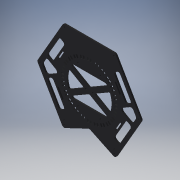
# Autodesk Inventor part: Bottom Plate
Saved by Autodesk Inventor 2017 (Build 210142000, 142)
## iProperties
Created: 2016-10-01
Part Number: Bottom Plate
Material: PVC, Unplasticized
Document SubType Name: Modeling
Designer: James Yelland
Density: 1.29 g/cm^3
Appearance: Smooth - White
Mass: 43.6601 g
Surface Area: 401.333 cm^2
Volume: 33.8451 cm^3
Author: James Yelland
Autodesk Inventor part; units mm, degrees
ref_plane "YZ Plane" through (0, 0, 0) normal (1, 0, 0) x (0, 1, 0)
ref_plane "XZ Plane" through (0, 0, 0) normal (0, 1, 0) x (-1, 0, 0)
ref_plane "XY Plane" through (0, 0, 0) normal (0, 0, 1) x (1, 0, 0)
sketch "Sketch1" plane through (0, 0, 0) normal (0, 1, 0) x (-1, 0, 0)
  line L0 (72.6878, -41.9663) -> (62.1878, -60.1529)
  line L1 (72.6878, -41.9663) -> (83.1878, -23.7798)
  line L2 (81.7237, -18.3157) -> (77.3936, -15.8157)
  line L3 (71.9295, -17.2797) -> (50.9295, -53.6529)
  line L4 (52.3936, -59.117) -> (56.7237, -61.617)
  arc A0 (56.7237, -61.617) -> (62.1878, -60.1529) centre (58.7237, -58.1529) ccw
  arc A1 (50.9295, -53.6529) -> (52.3936, -59.117) centre (54.3936, -55.6529) ccw
  arc A2 (77.3936, -15.8157) -> (71.9295, -17.2797) centre (75.3936, -19.2798) ccw
  arc A3 (83.1878, -23.7798) -> (81.7237, -18.3157) centre (79.7237, -21.7798) ccw
  line L5 (-72.6878, -41.9663) -> (-83.1878, -23.7798)
  line L6 (-72.6878, -41.9663) -> (-62.1878, -60.1529)
  line L7 (-56.7237, -61.617) -> (-52.3936, -59.117)
  line L8 (-50.9295, -53.6529) -> (-71.9294, -17.28)
  line L9 (-77.3936, -15.8157) -> (-81.7237, -18.3157)
  arc A4 (-81.7237, -18.3157) -> (-83.1878, -23.7798) centre (-79.7237, -21.7798) ccw
  arc A5 (-71.9294, -17.28) -> (-77.3936, -15.8157) centre (-75.3936, -19.2798) ccw
  arc A6 (-52.3936, -59.117) -> (-50.9295, -53.6529) centre (-54.3936, -55.6529) ccw
  arc A7 (-62.1878, -60.1529) -> (-56.7237, -61.617) centre (-58.7237, -58.1529) ccw
  line L10 (103.5566, -2.5) -> (54.8095, -86.9325)
  line L11 (-54.8095, -86.9325) -> (-103.5566, -2.5)
  line L12 (-103.5566, 2.5) -> (-53.9434, 88.4327)
  line L13 (-49.6132, 90.9327) -> (49.6132, 90.9327)
  line L14 (53.9434, 88.4327) -> (103.5566, 2.5)
  line L15 (2.1497, -66.9563) -> (48.3297, -88.9468)
  line L16 (-2.1497, -66.9563) -> (-48.3297, -88.9468)
  arc A8 (48.3297, -88.9468) -> (54.8095, -86.9325) centre (50.4794, -84.4325) ccw
  arc A9 (2.1497, -66.9563) -> (-2.1497, -66.9563) centre (0, -71.4706) ccw
  arc A10 (-54.8095, -86.9325) -> (-48.3297, -88.9468) centre (-50.4794, -84.4325) ccw
  arc A11 (-103.5566, 2.5) -> (-103.5566, -2.5) centre (-99.2265, 0) ccw
  arc A12 (-49.6132, 90.9327) -> (-53.9434, 88.4327) centre (-49.6132, 85.9327) ccw
  arc A13 (53.9434, 88.4327) -> (49.6132, 90.9327) centre (49.6132, 85.9327) ccw
  arc A14 (103.5566, -2.5) -> (103.5566, 2.5) centre (99.2265, 0) ccw
  circle A15 centre (49.6132, 85.9327) radius 1.6
  circle A16 centre (-49.6132, 85.9327) radius 1.6
  circle A17 centre (-99.2265, 0) radius 1.6
  circle A18 centre (99.2265, 0) radius 1.6
  arc A19 (-88.75, -10.8253) -> (-81.9199, -12.6554) centre (-84.4199, -8.3253) ccw
  arc A20 (-93.5566, 2.5) -> (-93.5566, -2.5) centre (-89.2265, 0) ccw
  arc A21 (81.9199, -12.6554) -> (88.75, -10.8253) centre (84.4199, -8.3253) ccw
  arc A22 (93.5566, -2.5) -> (93.5566, 2.5) centre (89.2265, 0) ccw
  line L17 (1.5, -53.75) -> (1.5, -56.75)
  line L18 (1.5, -56.75) -> (4.5, -56.75)
  line L19 (4.5, -56.75) -> (4.5, -50.75)
  line L20 (4.5, -50.75) -> (1.5, -50.75)
  line L21 (1.5, -50.75) -> (1.5, -53.75)
  line L22 (-1.5, -53.75) -> (-1.5, -56.75)
  line L23 (-1.5, -56.75) -> (-4.5, -56.75)
  line L24 (-1.5, -53.75) -> (-1.5, -53.75)
  line L25 (-1.5, -53.75) -> (-1.5, -50.75)
  line L26 (-1.5, -50.75) -> (-4.5, -50.75)
  line L27 (-4.5, -56.75) -> (-4.5, -50.75)
  line L28 (15.3604, -51.5303) -> (16.1369, -54.4281)
  line L29 (16.1369, -54.4281) -> (19.0346, -53.6516)
  line L30 (19.0346, -53.6516) -> (17.4817, -47.856)
  line L31 (17.4817, -47.856) -> (14.584, -48.6325)
  line L32 (14.584, -48.6325) -> (15.3604, -51.5303)
  line L33 (12.4626, -52.3067) -> (13.2391, -55.2045)
  line L34 (13.2391, -55.2045) -> (10.3413, -55.981)
  line L35 (12.4626, -52.3067) -> (11.6862, -49.409)
  line L36 (11.6862, -49.409) -> (8.7884, -50.1854)
  line L37 (10.3413, -55.981) -> (8.7884, -50.1854)
  line L38 (28.174, -45.7989) -> (29.674, -48.3969)
  line L39 (29.674, -48.3969) -> (32.2721, -46.8969)
  line L40 (32.2721, -46.8969) -> (29.2721, -41.7008)
  line L41 (29.2721, -41.7008) -> (26.674, -43.2008)
  line L42 (26.674, -43.2008) -> (28.174, -45.7989)
  line L43 (25.576, -47.2989) -> (27.076, -49.8969)
  line L44 (27.076, -49.8969) -> (24.4779, -51.3969)
  line L45 (25.576, -47.2989) -> (24.076, -44.7008)
  line L46 (24.076, -44.7008) -> (21.4779, -46.2008)
  line L47 (24.4779, -51.3969) -> (21.4779, -46.2008)
  line L48 (39.0676, -36.9463) -> (41.189, -39.0676)
  line L49 (41.189, -39.0676) -> (43.3103, -36.9463)
  line L50 (43.3103, -36.9463) -> (39.0676, -32.7037)
  line L51 (39.0676, -32.7037) -> (36.9463, -34.825)
  line L52 (36.9463, -34.825) -> (39.0676, -36.9463)
  line L53 (36.9463, -39.0676) -> (39.0676, -41.189)
  line L54 (39.0676, -41.189) -> (36.9463, -43.3103)
  line L55 (36.9463, -39.0676) -> (34.825, -36.9463)
  line L56 (34.825, -36.9463) -> (32.7037, -39.0676)
  line L57 (36.9463, -43.3103) -> (32.7037, -39.0676)
  line L58 (47.2989, -25.576) -> (49.8969, -27.076)
  line L59 (49.8969, -27.076) -> (51.3969, -24.4779)
  line L60 (51.3969, -24.4779) -> (46.2008, -21.4779)
  line L61 (46.2008, -21.4779) -> (44.7008, -24.076)
  line L62 (44.7008, -24.076) -> (47.2989, -25.576)
  line L63 (45.7989, -28.174) -> (48.3969, -29.674)
  line L64 (48.3969, -29.674) -> (46.8969, -32.2721)
  line L65 (45.7989, -28.174) -> (43.2008, -26.674)
  line L66 (43.2008, -26.674) -> (41.7008, -29.2721)
  line L67 (46.8969, -32.2721) -> (41.7008, -29.2721)
  line L68 (52.3067, -12.4626) -> (55.2045, -13.2391)
  line L69 (55.2045, -13.2391) -> (55.981, -10.3413)
  line L70 (55.981, -10.3413) -> (50.1854, -8.7884)
  line L71 (50.1854, -8.7884) -> (49.409, -11.6862)
  line L72 (49.409, -11.6862) -> (52.3067, -12.4626)
  line L73 (51.5303, -15.3604) -> (54.4281, -16.1369)
  line L74 (54.4281, -16.1369) -> (53.6516, -19.0346)
  line L75 (51.5303, -15.3604) -> (48.6325, -14.584)
  line L76 (48.6325, -14.584) -> (47.856, -17.4817)
  line L77 (53.6516, -19.0346) -> (47.856, -17.4817)
  line L78 (53.75, 1.5) -> (56.75, 1.5)
  line L79 (56.75, 1.5) -> (56.75, 4.5)
  line L80 (56.75, 4.5) -> (50.75, 4.5)
  line L81 (50.75, 4.5) -> (50.75, 1.5)
  line L82 (50.75, 1.5) -> (53.75, 1.5)
  line L83 (53.75, -1.5) -> (56.75, -1.5)
  line L84 (56.75, -1.5) -> (56.75, -4.5)
  line L85 (53.75, -1.5) -> (50.75, -1.5)
  line L86 (50.75, -1.5) -> (50.75, -4.5)
  line L87 (56.75, -4.5) -> (50.75, -4.5)
  line L88 (51.5303, 15.3604) -> (54.4281, 16.1369)
  line L89 (54.4281, 16.1369) -> (53.6516, 19.0346)
  line L90 (53.6516, 19.0346) -> (47.856, 17.4817)
  line L91 (47.856, 17.4817) -> (48.6325, 14.584)
  line L92 (48.6325, 14.584) -> (51.5303, 15.3604)
  line L93 (52.3067, 12.4626) -> (55.2045, 13.2391)
  line L94 (55.2045, 13.2391) -> (55.981, 10.3413)
  line L95 (52.3067, 12.4626) -> (49.409, 11.6862)
  line L96 (49.409, 11.6862) -> (50.1854, 8.7884)
  line L97 (55.981, 10.3413) -> (50.1854, 8.7884)
  line L98 (45.7989, 28.174) -> (48.3969, 29.674)
  line L99 (48.3969, 29.674) -> (46.8969, 32.2721)
  line L100 (46.8969, 32.2721) -> (41.7008, 29.2721)
  line L101 (41.7008, 29.2721) -> (43.2008, 26.674)
  line L102 (43.2008, 26.674) -> (45.7989, 28.174)
  line L103 (47.2989, 25.576) -> (49.8969, 27.076)
  line L104 (49.8969, 27.076) -> (51.3969, 24.4779)
  line L105 (47.2989, 25.576) -> (44.7008, 24.076)
  line L106 (44.7008, 24.076) -> (46.2008, 21.4779)
  line L107 (51.3969, 24.4779) -> (46.2008, 21.4779)
  line L108 (36.9463, 39.0676) -> (39.0676, 41.189)
  line L109 (39.0676, 41.189) -> (36.9463, 43.3103)
  line L110 (36.9463, 43.3103) -> (32.7037, 39.0676)
  line L111 (32.7037, 39.0676) -> (34.825, 36.9463)
  line L112 (34.825, 36.9463) -> (36.9463, 39.0676)
  line L113 (39.0676, 36.9463) -> (41.189, 39.0676)
  line L114 (41.189, 39.0676) -> (43.3103, 36.9463)
  line L115 (39.0676, 36.9463) -> (36.9463, 34.825)
  line L116 (36.9463, 34.825) -> (39.0676, 32.7037)
  line L117 (43.3103, 36.9463) -> (39.0676, 32.7037)
  line L118 (25.576, 47.2989) -> (27.076, 49.8969)
  line L119 (27.076, 49.8969) -> (24.4779, 51.3969)
  line L120 (24.4779, 51.3969) -> (21.4779, 46.2008)
  line L121 (21.4779, 46.2008) -> (24.076, 44.7008)
  line L122 (24.076, 44.7008) -> (25.576, 47.2989)
  line L123 (28.174, 45.7989) -> (29.674, 48.3969)
  line L124 (29.674, 48.3969) -> (32.2721, 46.8969)
  line L125 (28.174, 45.7989) -> (26.674, 43.2008)
  line L126 (26.674, 43.2008) -> (29.2721, 41.7008)
  line L127 (32.2721, 46.8969) -> (29.2721, 41.7008)
  line L128 (12.4626, 52.3067) -> (13.2391, 55.2045)
  line L129 (13.2391, 55.2045) -> (10.3413, 55.981)
  line L130 (10.3413, 55.981) -> (8.7884, 50.1854)
  line L131 (8.7884, 50.1854) -> (11.6862, 49.409)
  line L132 (11.6862, 49.409) -> (12.4626, 52.3067)
  line L133 (15.3604, 51.5303) -> (16.1369, 54.4281)
  line L134 (16.1369, 54.4281) -> (19.0346, 53.6516)
  line L135 (15.3604, 51.5303) -> (14.584, 48.6325)
  line L136 (14.584, 48.6325) -> (17.4817, 47.856)
  line L137 (19.0346, 53.6516) -> (17.4817, 47.856)
  line L138 (-1.5, 53.75) -> (-1.5, 56.75)
  line L139 (-1.5, 56.75) -> (-4.5, 56.75)
  line L140 (-4.5, 56.75) -> (-4.5, 50.75)
  line L141 (-4.5, 50.75) -> (-1.5, 50.75)
  line L142 (-1.5, 50.75) -> (-1.5, 53.75)
  line L143 (1.5, 53.75) -> (1.5, 56.75)
  line L144 (1.5, 56.75) -> (4.5, 56.75)
  line L145 (1.5, 53.75) -> (1.5, 50.75)
  line L146 (1.5, 50.75) -> (4.5, 50.75)
  line L147 (4.5, 56.75) -> (4.5, 50.75)
  line L148 (-15.3604, 51.5303) -> (-16.1369, 54.4281)
  line L149 (-16.1369, 54.4281) -> (-19.0346, 53.6516)
  line L150 (-19.0346, 53.6516) -> (-17.4817, 47.856)
  line L151 (-17.4817, 47.856) -> (-14.584, 48.6325)
  line L152 (-14.584, 48.6325) -> (-15.3604, 51.5303)
  line L153 (-12.4626, 52.3067) -> (-13.2391, 55.2045)
  line L154 (-13.2391, 55.2045) -> (-10.3413, 55.981)
  line L155 (-12.4626, 52.3067) -> (-11.6862, 49.409)
  line L156 (-11.6862, 49.409) -> (-8.7884, 50.1854)
  line L157 (-10.3413, 55.981) -> (-8.7884, 50.1854)
  line L158 (-28.174, 45.7989) -> (-29.674, 48.3969)
  line L159 (-29.674, 48.3969) -> (-32.2721, 46.8969)
  line L160 (-32.2721, 46.8969) -> (-29.2721, 41.7008)
  line L161 (-29.2721, 41.7008) -> (-26.674, 43.2008)
  line L162 (-26.674, 43.2008) -> (-28.174, 45.7989)
  line L163 (-25.576, 47.2989) -> (-27.076, 49.8969)
  line L164 (-27.076, 49.8969) -> (-24.4779, 51.3969)
  line L165 (-25.576, 47.2989) -> (-24.076, 44.7008)
  line L166 (-24.076, 44.7008) -> (-21.4779, 46.2008)
  line L167 (-24.4779, 51.3969) -> (-21.4779, 46.2008)
  line L168 (-39.0676, 36.9463) -> (-41.189, 39.0676)
  line L169 (-41.189, 39.0676) -> (-43.3103, 36.9463)
  line L170 (-43.3103, 36.9463) -> (-39.0676, 32.7037)
  line L171 (-39.0676, 32.7037) -> (-36.9463, 34.825)
  line L172 (-36.9463, 34.825) -> (-39.0676, 36.9463)
  line L173 (-36.9463, 39.0676) -> (-39.0676, 41.189)
  line L174 (-39.0676, 41.189) -> (-36.9463, 43.3103)
  line L175 (-36.9463, 39.0676) -> (-34.825, 36.9463)
  line L176 (-34.825, 36.9463) -> (-32.7037, 39.0676)
  line L177 (-36.9463, 43.3103) -> (-32.7037, 39.0676)
  line L178 (-47.2989, 25.576) -> (-49.8969, 27.076)
  line L179 (-49.8969, 27.076) -> (-51.3969, 24.4779)
  line L180 (-51.3969, 24.4779) -> (-46.2008, 21.4779)
  line L181 (-46.2008, 21.4779) -> (-44.7008, 24.076)
  line L182 (-44.7008, 24.076) -> (-47.2989, 25.576)
  line L183 (-45.7989, 28.174) -> (-48.3969, 29.674)
  line L184 (-48.3969, 29.674) -> (-46.8969, 32.2721)
  line L185 (-45.7989, 28.174) -> (-43.2008, 26.674)
  line L186 (-43.2008, 26.674) -> (-41.7008, 29.2721)
  line L187 (-46.8969, 32.2721) -> (-41.7008, 29.2721)
  line L188 (-52.3067, 12.4626) -> (-55.2045, 13.2391)
  line L189 (-55.2045, 13.2391) -> (-55.981, 10.3413)
  line L190 (-55.981, 10.3413) -> (-50.1854, 8.7884)
  line L191 (-50.1854, 8.7884) -> (-49.409, 11.6862)
  line L192 (-49.409, 11.6862) -> (-52.3067, 12.4626)
  line L193 (-51.5303, 15.3604) -> (-54.4281, 16.1369)
  line L194 (-54.4281, 16.1369) -> (-53.6516, 19.0346)
  line L195 (-51.5303, 15.3604) -> (-48.6325, 14.584)
  line L196 (-48.6325, 14.584) -> (-47.856, 17.4817)
  line L197 (-53.6516, 19.0346) -> (-47.856, 17.4817)
  line L198 (-53.75, -1.5) -> (-56.75, -1.5)
  line L199 (-56.75, -1.5) -> (-56.75, -4.5)
  line L200 (-56.75, -4.5) -> (-50.75, -4.5)
  line L201 (-50.75, -4.5) -> (-50.75, -1.5)
  line L202 (-50.75, -1.5) -> (-53.75, -1.5)
  line L203 (-53.75, 1.5) -> (-56.75, 1.5)
  line L204 (-56.75, 1.5) -> (-56.75, 4.5)
  line L205 (-53.75, 1.5) -> (-50.75, 1.5)
  line L206 (-50.75, 1.5) -> (-50.75, 4.5)
  line L207 (-56.75, 4.5) -> (-50.75, 4.5)
  line L208 (-51.5303, -15.3604) -> (-54.4281, -16.1369)
  line L209 (-54.4281, -16.1369) -> (-53.6516, -19.0346)
  line L210 (-53.6516, -19.0346) -> (-47.856, -17.4817)
  line L211 (-47.856, -17.4817) -> (-48.6325, -14.584)
  line L212 (-48.6325, -14.584) -> (-51.5303, -15.3604)
  line L213 (-52.3067, -12.4626) -> (-55.2045, -13.2391)
  line L214 (-55.2045, -13.2391) -> (-55.981, -10.3413)
  line L215 (-52.3067, -12.4626) -> (-49.409, -11.6862)
  line L216 (-49.409, -11.6862) -> (-50.1854, -8.7884)
  line L217 (-55.981, -10.3413) -> (-50.1854, -8.7884)
  line L218 (-45.7989, -28.174) -> (-48.3969, -29.674)
  line L219 (-48.3969, -29.674) -> (-46.8969, -32.2721)
  line L220 (-46.8969, -32.2721) -> (-41.7008, -29.2721)
  line L221 (-41.7008, -29.2721) -> (-43.2008, -26.674)
  line L222 (-43.2008, -26.674) -> (-45.7989, -28.174)
  line L223 (-47.2989, -25.576) -> (-49.8969, -27.076)
  line L224 (-49.8969, -27.076) -> (-51.3969, -24.4779)
  line L225 (-47.2989, -25.576) -> (-44.7008, -24.076)
  line L226 (-44.7008, -24.076) -> (-46.2008, -21.4779)
  line L227 (-51.3969, -24.4779) -> (-46.2008, -21.4779)
  line L228 (-36.9463, -39.0676) -> (-39.0676, -41.189)
  line L229 (-39.0676, -41.189) -> (-36.9463, -43.3103)
  line L230 (-36.9463, -43.3103) -> (-32.7037, -39.0676)
  line L231 (-32.7037, -39.0676) -> (-34.825, -36.9463)
  line L232 (-34.825, -36.9463) -> (-36.9463, -39.0676)
  line L233 (-39.0676, -36.9463) -> (-41.189, -39.0676)
  line L234 (-41.189, -39.0676) -> (-43.3103, -36.9463)
  line L235 (-39.0676, -36.9463) -> (-36.9463, -34.825)
  line L236 (-36.9463, -34.825) -> (-39.0676, -32.7037)
  line L237 (-43.3103, -36.9463) -> (-39.0676, -32.7037)
  line L238 (-25.576, -47.2989) -> (-27.076, -49.8969)
  line L239 (-27.076, -49.8969) -> (-24.4779, -51.3969)
  line L240 (-24.4779, -51.3969) -> (-21.4779, -46.2008)
  line L241 (-21.4779, -46.2008) -> (-24.076, -44.7008)
  line L242 (-24.076, -44.7008) -> (-25.576, -47.2989)
  line L243 (-28.174, -45.7989) -> (-29.674, -48.3969)
  line L244 (-29.674, -48.3969) -> (-32.2721, -46.8969)
  line L245 (-28.174, -45.7989) -> (-26.674, -43.2008)
  line L246 (-26.674, -43.2008) -> (-29.2721, -41.7008)
  line L247 (-32.2721, -46.8969) -> (-29.2721, -41.7008)
  line L248 (-12.4626, -52.3067) -> (-13.2391, -55.2045)
  line L249 (-13.2391, -55.2045) -> (-10.3413, -55.981)
  line L250 (-10.3413, -55.981) -> (-8.7884, -50.1854)
  line L251 (-8.7884, -50.1854) -> (-11.6862, -49.409)
  line L252 (-11.6862, -49.409) -> (-12.4626, -52.3067)
  line L253 (-15.3604, -51.5303) -> (-16.1369, -54.4281)
  line L254 (-16.1369, -54.4281) -> (-19.0346, -53.6516)
  line L255 (-15.3604, -51.5303) -> (-14.584, -48.6325)
  line L256 (-14.584, -48.6325) -> (-17.4817, -47.856)
  line L257 (-19.0346, -53.6516) -> (-17.4817, -47.856)
  arc A23 (-83.1878, 23.7798) -> (-81.7237, 18.3157) centre (-79.7237, 21.7798) ccw
  line L258 (-81.7237, 18.3157) -> (-77.3936, 15.8157)
  arc A24 (-77.3936, 15.8157) -> (-71.9295, 17.2798) centre (-75.3936, 19.2798) ccw
  line L259 (-72.6878, 41.9663) -> (-83.1878, 23.7798)
  line L260 (-71.9295, 17.2798) -> (-50.9296, 53.6527)
  line L261 (-72.6878, 41.9663) -> (-62.1878, 60.1529)
  arc A25 (-56.7237, 61.617) -> (-62.1878, 60.1529) centre (-58.7237, 58.1529) ccw
  line L262 (-52.3936, 59.117) -> (-56.7237, 61.617)
  arc A26 (-50.9296, 53.6527) -> (-52.3936, 59.117) centre (-54.3936, 55.6529) ccw
  arc A27 (-81.9199, 12.6554) -> (-88.75, 10.8253) centre (-84.4199, 8.3253) ccw
  arc A28 (62.1878, 60.1529) -> (56.7237, 61.6169) centre (58.7237, 58.1528) ccw
  line L263 (56.7237, 61.6169) -> (52.3936, 59.1169)
  arc A29 (52.3936, 59.1169) -> (50.9295, 53.6528) centre (54.3936, 55.6528) ccw
  line L264 (72.6878, 41.9663) -> (62.1878, 60.1529)
  line L265 (50.9295, 53.6528) -> (71.9295, 17.2798)
  line L266 (72.6878, 41.9663) -> (83.1878, 23.7798)
  arc A30 (81.7237, 18.3157) -> (83.1878, 23.7798) centre (79.7237, 21.7798) ccw
  line L267 (77.3936, 15.8157) -> (81.7237, 18.3157)
  arc A31 (71.9295, 17.2798) -> (77.3936, 15.8157) centre (75.3936, 19.2798) ccw
  arc A32 (88.75, 10.8253) -> (81.9199, 12.6554) centre (84.4199, 8.3253) ccw
  arc A33 (67.5, 4.3301) -> (67.5, -4.3301) centre (70, 0) ccw
  arc A34 (-67.5, -4.3301) -> (-67.5, 4.3301) centre (-70, 0) ccw
  line L268 (-67.5, -4.3301) -> (-81.9199, -12.6554)
  line L269 (-88.75, -10.8253) -> (-93.5566, -2.5)
  line L270 (-93.5566, 2.5) -> (-88.75, 10.8253)
  line L271 (-81.9199, 12.6554) -> (-67.5, 4.3301)
  line L272 (81.9199, 12.6554) -> (67.5, 4.3301)
  line L273 (67.5, -4.3301) -> (81.9199, -12.6554)
  line L274 (88.75, -10.8253) -> (93.5566, -2.5)
  line L275 (93.5566, 2.5) -> (88.75, 10.8253)
  line L276 (0, 30) -> (-31.225, 30)
  line L277 (0, 30) -> (31.225, 30)
  line L278 (0, -30) -> (-31.225, -30)
  line L279 (0, -30) -> (31.225, -30)
  arc A35 (42.1141, -15.8557) -> (42.1141, 15.8557) centre (0, 0) ccw
  arc A36 (-42.1141, 15.8558) -> (-42.1141, -15.8558) centre (0, 0) ccw
  arc A37 (34.525, 28.7563) -> (31.225, 30) centre (31.225, 25) ccw
  arc A38 (-31.225, 30) -> (-34.525, 28.7563) centre (-31.225, 25) ccw
  arc A39 (-34.525, -28.7563) -> (-31.225, -30) centre (-31.225, -25) ccw
  arc A40 (31.225, -30) -> (34.525, -28.7563) centre (31.225, -25) ccw
  circle A41 centre (22.6343, 38) radius 1.6
  circle A42 centre (-22.6343, 38) radius 1.6
  circle A43 centre (-22.6343, -38) radius 1.6
  circle A44 centre (22.6343, -38) radius 1.6
  line L280 (61.4295, 35.4663) -> (63.9295, 31.1362)
  line L281 (39.2424, -16.8831) -> (13, -1.7321)
  line L282 (39.2424, 16.8831) -> (13, 1.7321)
  line L283 (34.205, 25.5218) -> (1, 6.3509)
  line L284 (-1, 6.3509) -> (-34.205, 25.5218)
  line L285 (-39.2423, 16.8832) -> (-12.9998, 1.7321)
  line L286 (-12.9998, -1.7321) -> (-39.2423, -16.8832)
  line L287 (-34.205, -25.5218) -> (-1, -6.3509)
  line L288 (1, -6.3509) -> (34.205, -25.5218)
  arc A45 (-1, 6.3509) -> (1, 6.3509) centre (0, 8.0829) ccw
  arc A46 (-12.9998, -1.7321) -> (-12.9998, 1.7321) centre (-13.9998, 0) ccw
  arc A47 (1, -6.3509) -> (-1, -6.3509) centre (0, -8.0829) ccw
  arc A48 (13, 1.7321) -> (13, -1.7321) centre (14, 0) ccw
  arc A49 (39.2424, -16.8831) -> (42.1141, -15.8557) centre (40.2424, -15.151) ccw
  arc A50 (34.525, -28.7563) -> (34.205, -25.5218) centre (33.205, -27.2538) ccw
  arc A51 (-42.1141, -15.8558) -> (-39.2423, -16.8832) centre (-40.2423, -15.1511) ccw
  arc A52 (-34.205, -25.5218) -> (-34.525, -28.7563) centre (-33.205, -27.2538) ccw
  arc A53 (-39.2423, 16.8832) -> (-42.1141, 15.8558) centre (-40.2423, 15.1511) ccw
  arc A54 (-34.525, 28.7563) -> (-34.205, 25.5218) centre (-33.205, 27.2538) ccw
  arc A55 (42.1141, 15.8557) -> (39.2424, 16.8831) centre (40.2424, 15.151) ccw
  arc A56 (34.205, 25.5218) -> (34.525, 28.7563) centre (33.205, 27.2538) ccw
  circle A57 centre (7, 0) radius 1.6
  circle A58 centre (-7, 0) radius 1.6
  circle A59 centre (50.4794, -84.4325) radius 1.45
  circle A60 centre (50.4794, -76.4325) radius 1.45
  circle A61 centre (-50.4794, -84.4325) radius 1.45
  circle A62 centre (-50.4794, -76.4325) radius 1.45
  line L289 (59.0479, -34.0913) -> (53.9979, -42.8382)
  line L290 (53.9979, -42.8382) -> (51.2266, -41.2382)
  line L291 (51.2266, -41.2382) -> (61.3266, -23.7445)
  line L292 (61.3266, -23.7445) -> (64.0979, -25.3445)
  line L293 (64.0979, -25.3445) -> (59.0479, -34.0913)
  line L294 (59.0479, 34.0913) -> (53.9979, 42.8382)
  line L295 (53.9979, 42.8382) -> (51.2266, 41.2382)
  line L296 (51.2266, 41.2382) -> (61.3266, 23.7445)
  line L297 (61.3266, 23.7445) -> (64.0979, 25.3445)
  line L298 (64.0979, 25.3445) -> (59.0479, 34.0913)
  line L299 (-59.0479, -34.0913) -> (-53.9979, -42.8382)
  line L300 (-53.9979, -42.8382) -> (-51.2266, -41.2382)
  line L301 (-51.2266, -41.2382) -> (-61.3266, -23.7445)
  line L302 (-61.3266, -23.7445) -> (-64.0979, -25.3445)
  line L303 (-64.0979, -25.3445) -> (-59.0479, -34.0913)
  line L304 (-51.2266, 41.2382) -> (-61.3266, 23.7445)
  line L305 (-64.0979, 25.3445) -> (-59.0479, 34.0913)
  line L306 (-61.3266, 23.7445) -> (-64.0979, 25.3445)
  line L307 (-53.9979, 42.8382) -> (-51.2266, 41.2382)
  line L308 (-59.0479, 34.0913) -> (-53.9979, 42.8382)
  point P0 (60.1878, -63.617)
  point P1 (85.1878, -20.3157)
  point P2 (73.9295, -13.8157)
  point P3 (48.9295, -57.117)
  point P4 (-85.1878, -20.3157)
  point P5 (-60.1878, -63.617)
  point P6 (-48.9295, -57.117)
  point P7 (-73.9295, -13.8157)
  point P8 (105, 0)
  point P9 (52.5, -90.9327)
  point P10 (-105, 0)
  point P11 (-52.5, 90.9327)
  point P12 (52.5, 90.9327)
  point P13 (-86.25, -15.1554)
  point P14 (60, 0)
  point P15 (-60, 0)
  point P16 (-73.9295, 13.8157)
  point P17 (-85.1878, 20.3157)
  point P18 (-48.9295, 57.117)
  point P19 (-60.1878, 63.617)
  point P20 (-60, 0)
  point P21 (48.9295, 57.1169)
  point P22 (60.1878, 63.6169)
  point P23 (73.9295, 13.8157)
  point P24 (85.1878, 20.3157)
  point P25 (60, 0)
  point P26 (-33.541, 30)
  point P27 (33.541, 30)
  point P28 (-33.541, -30)
  point P29 (33.541, -30)
  point P30 (41.2298, -18.0305)
  point P31 (41.2298, 18.0305)
  point P32 (-41.2298, 18.0306)
  point P33 (-41.2298, -18.0306)
  dimension "d11" = 360
  dimension "d30" = 360
  dimension "d114" = 360
  constraints: 618 end point, 106 point on circle, 80 point on line, 63 centre point, 5 coincident, 1 midpoint, 1 other
extrude "Extrusion1" add sketch "Sketch1" along normal blind 3
body "Solid1"
